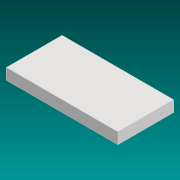
# Autodesk Inventor part: 汽缸3
Saved by Autodesk Inventor 2020 (Build 240168000, 168)
## iProperties
Created: 2023-03-16
Part Number: 汽缸3
Material: 一般
Document SubType Name: Modeling
Designer: ASUS
Density: 1 g/cm^3
Appearance: 預設
Author: ASUS
Autodesk Inventor part; units mm, degrees
ref_plane "YZ Plane" through (0, 0, 0) normal (1, 0, 0) x (0, 1, 0)
ref_plane "XZ Plane" through (0, 0, 0) normal (0, 1, 0) x (-1, 0, 0)
ref_plane "XY Plane" through (0, 0, 0) normal (0, 0, 1) x (1, 0, 0)
sketch "草圖1" plane through (0, 0, 0) normal (0, 1, 0) x (-1, 0, 0)
  line L0 (-50, 0) -> (50, 0)
  line L1 (50, 0) -> (50, 50)
  line L2 (50, 50) -> (-50, 50)
  line L3 (-50, 50) -> (-50, 0)
  point P0 (0, 0)
  point P1 (0, 0)
  dimension "d0" = 50
  dimension "d1" = 100
  constraints: 8 end point, 2 parallel, 1 coincident, 1 horizontal, 1 midpoint, 1 perpendicular
  measures "d0" distance of L0.end L1.end
  measures "d1" distance of L1.end L2.end
extrude "擠出1" add sketch "草圖1" along normal mid plane 50
